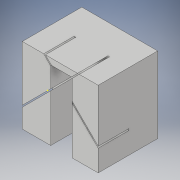
# Autodesk Inventor part: crosspiecejig
Saved by Autodesk Inventor 2018 (Build 220112000, 112)
## iProperties
Created: 2019-02-01
Part Number: crosspiecejig
Material: Generic
Document SubType Name: Modeling
Designer: F8PLTW
Density: 1 g/cm^3
Appearance: Default
Author: F8PLTW
Autodesk Inventor part; units mm, degrees
ref_plane "YZ Plane" through (0, 0, 0) normal (1, 0, 0) x (0, 1, 0)
ref_plane "XZ Plane" through (0, 0, 0) normal (0, 1, 0) x (-1, 0, 0)
ref_plane "XY Plane" through (0, 0, 0) normal (0, 0, 1) x (1, 0, 0)
sketch "Sketch1" plane through (0, 0, 0) normal (0, 0, 1) x (1, 0, 0)
  line L0 (-4.2367, 4.9428) -> (8.4633, 4.9428)
  line L1 (8.4633, 4.9428) -> (8.4633, -7.7572)
  line L2 (8.4633, -7.7572) -> (-4.2367, -7.7572)
  line L3 (-4.2367, -7.7572) -> (-4.2367, 4.9428)
  point P0 (0, 0)
  dimension "d0" = 12.7
  dimension "d1" = 12.7
  constraints: 8 end point, 2 parallel, 1 horizontal, 1 perpendicular
  measures "d0" distance of L1.end L2.end
  measures "d1" distance of L0.end L1.end
extrude "Extrusion1" add sketch "Sketch1" along normal blind 6.35
sketch "Sketch2" plane through (0, 0, 6.35) normal (0, 0, 1) x (1, 0, 0)
  line L0 (-4.2367, -7.7572) -> (8.4633, -7.7572) projected
  line L1 (0.5135, -7.7572) -> (4.1203, -7.7572)
  line L2 (4.1203, -7.7572) -> (4.1203, 4.9428)
  line L3 (8.4633, 4.9428) -> (-4.2367, 4.9428) projected
  line L4 (4.1203, 4.9428) -> (0.5135, 4.9428)
  line L5 (0.5135, -7.7572) -> (0.5135, 4.9428)
  line L6 (0.5135, 4.9428) -> (-4.2367, 4.9428)
  line L7 (-4.2367, 4.9428) -> (-4.2367, -7.7572)
  line L8 (-4.2367, -7.7572) -> (0.5135, -7.7572)
  line L9 (0.5135, -7.7572) -> (0.5135, 4.9428)
  line L10 (4.1203, 4.9428) -> (8.4633, 4.9428)
  line L11 (8.4633, 4.9428) -> (8.4633, -7.7572)
  line L12 (8.4633, -7.7572) -> (4.1203, -7.7572)
  line L13 (4.1203, -7.7572) -> (4.1203, 4.9428)
  point P0 (0, 0)
  dimension "d4" = 3.6068
  constraints: 24 end point, 4 parallel, 4 perpendicular, 4 point on line, 2 horizontal
  measures "d4" distance of L1.start L1.end
extrude "Extrusion2" add sketch "Sketch2" along normal blind 3.6068 contours L7 L3 L5 L0 | L2 L3 L11 L0
sketch "Sketch3" plane through (0, 0, 6.35) normal (0, 0, 1) x (1, 0, 0)
  line L0 (4.1203, 4.9428) -> (0.5135, 4.9428) projected
  line L1 (4.1203, 4.9428) -> (4.1203, -7.7572) projected
  line L2 (0.5135, 4.9428) -> (4.1203, 4.9428)
  line L3 (4.1203, 4.9428) -> (4.1203, 3.9157)
  line L4 (4.1203, 3.9157) -> (0.5135, 3.9157)
  line L5 (0.5135, 3.9157) -> (0.5135, 4.9428)
  point P0 (0, 0)
  constraints: 8 end point, 2 parallel, 1 horizontal, 1 perpendicular, 1 point on line
extrude "Extrusion3" add sketch "Sketch3" along normal blind 3.6068
sketch "Sketch4" plane through (0, 0, 9.9568) normal (0, 0, 1) x (1, 0, 0)
  line L0 (0.5135, -7.7572) -> (0.5135, 3.9157) projected
  line L1 (0.5135, 3.9157) -> (11.3187, 3.9157) construction
  line L2 (4.1203, -7.7572) -> (4.1203, 3.9157) projected
  line L3 (-4.2367, 4.9428) -> (-4.2367, -7.7572) projected
  line L4 (8.4633, 4.9428) -> (-4.2367, 4.9428) projected
  line L5 (8.4633, -7.7572) -> (8.4633, 4.9428) projected
  line L6 (8.4633, -6.0235) -> (8.4633, -1.9417)
  line L7 (-4.2367, -2.4282) -> (-4.2367, -6.55)
  line L8 (8.4633, -4.1258) -> (8.4633, -3.8394)
  line L9 (-4.2367, -4.6399) -> (-4.2367, -4.3516)
  line L10 (0.5135, 3.9157) -> (8.4633, -4.0341) construction
  line L11 (0.5135, 3.9157) -> (11.7563, 3.9157) construction
  line L12 (4.1203, 3.9157) -> (-3.8295, -4.0341) construction
  line L13 (4.1203, 3.9157) -> (15.3631, 3.9157) construction
  line L14 (4.1203, 3.9157) -> (5.1474, 4.9428) construction
  line L15 (0.5135, 3.9157) -> (-0.5135, 4.9428) construction
  line L16 (-0.5854, 4.8709) -> (8.4633, -4.1778)
  line L17 (8.4633, -3.8904) -> (0.0898, 4.4832)
  line L18 (0.0898, 4.4832) -> (-0.3699, 4.9428)
  line L19 (-0.5854, 4.8709) -> (-0.6572, 4.9428)
  line L20 (-3.6868, -4.0351) -> (5.3778, 5.0295)
  line L21 (4.5252, 4.4643) -> (-4.2367, -4.2976)
  line L22 (-3.6868, -4.0351) -> (-4.2367, -4.585)
  line L23 (-4.2367, -4.2976) -> (-4.2367, -4.585)
  line L24 (5.3778, 5.0295) -> (5.0904, 5.0295)
  line L25 (5.0904, 5.0295) -> (4.5252, 4.4643)
  point P0 (0, 0)
  dimension "d22" = 45
  dimension "d23" = 135
  dimension "d24" = 0.2032
  dimension "d25" = 0.2032
  constraints: 42 end point, 17 point on line, 6 collinear, 4 horizontal, 3 parallel, 2 equal length, 1 perpendicular, 1 vertical, 2 other
  measures "d22" angle of L10 L11
  measures "d23" angle of L12 L13
  measures "d24" distance between parallel lines of L16 L17
  measures "d25" distance between parallel lines of L21 L20
extrude "Extrusion7" cut sketch "Sketch4" against normal blind 5.08 contours L20 L22 L3 L21 L0 | L0 L21 L16 L20 | L20 L17 L2 L16 | L16 L21 L17 L20 | L16 L19 L4 L18 L17 L21 | L2 L17 L5 L16 | L17 L21 L25 L4 L20 | L4 L25 L24 L20
sketch "Sketch7" plane through (0, 0, 9.9568) normal (0, 0, 1) x (1, 0, 0)
  point P0 (0, 0)
body "Solid1"
